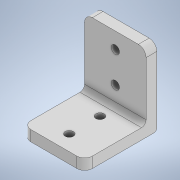
# Autodesk Inventor part: angulares
Saved by Autodesk Inventor 2022 (Build 260153000, 153)
## iProperties
Created: 2022-02-04
Part Number: angulares
Material: Generic
Document SubType Name: Modeling
Designer: Home
Density: 1 g/cm^3
Appearance: Default
Author: Home
Autodesk Inventor part; units mm, degrees
ref_plane "YZ Plane" through (0, 0, 0) normal (1, 0, 0) x (0, 1, 0)
ref_plane "XZ Plane" through (0, 0, 0) normal (0, 1, 0) x (-1, 0, 0)
ref_plane "XY Plane" through (0, 0, 0) normal (0, 0, 1) x (1, 0, 0)
sketch "Sketch1" plane through (0, 0, 0) normal (0, 1, 0) x (-1, 0, 0)
  line L0 (20, -20) -> (-20, -20)
  line L1 (-20, -20) -> (-20, 20)
  line L2 (-20, 20) -> (20, 20)
  line L3 (20, 20) -> (20, -20)
  line L4 (20, -20) -> (-20, 20) construction
  line L5 (-20, -20) -> (20, 20) construction
  point P0 (0, 0)
  dimension "d0" = 40
  dimension "d1" = 40
  constraints: 12 end point, 2 midpoint, 2 parallel, 1 horizontal, 1 perpendicular
  measures "d0" distance of L0.end L1.end
  measures "d1" distance of L0.start L0.end
extrude "Extrusion1" add sketch "Sketch1" along normal blind 7
sketch "Sketch2" plane through (0, 7, 0) normal (0, 1, 0) x (1, 0, 0)
  line L0 (-20, -20) -> (20, -20) projected
  point P0 (0, 0)
  point P1 (0, -10)
  point P2 (0, 10)
  dimension "d4" = 20
  dimension "d5" = 10
  constraints: 2 vertical alignment
  measures "d4" distance of point (0, 10) point (0, -10)
  measures "d5" distance from line of point (0, -10) L0
sketch "Sketch3" plane through (20, 0, -20) normal (0, 0, -1) x (-1, 0, 0)
  line L0 (0, 0) -> (0, 7) projected
  line L1 (0, 0) -> (40, 0)
  line L2 (40, 0) -> (40, 50)
  line L3 (40, 50) -> (0, 50)
  line L4 (0, 50) -> (0, 0)
  point P0 (20, 0)
  dimension "d14" = 50
  dimension "d15" = 40
  constraints: 8 end point, 2 parallel, 1 horizontal, 1 perpendicular
  measures "d14" distance of L3.end L0.start
  measures "d15" distance of L0.start L1.end
extrude "Extrusion2" add sketch "Sketch3" along normal blind 7
fillet "Fillet2" radius 3 1 edges at (0, 7, -20)
fillet "Fillet2" radius 5 4 edges at (-20, 50, -23.5) (20, 50, -23.5) (-20, 3.5, 20) (20, 3.5, 20)
fillet "Fillet2" radius 2 1 edges at (0, 0, -27)
sketch "Sketch4" plane through (20, 0, -20) normal (0, 0, 1) x (1, 0, 0)
  line L0 (-35, 0) -> (-5, 0) projected
  line L1 (-40, 7) -> (0, 7) projected
  point P0 (-20, 0)
  point P1 (-20, 39.5)
  point P2 (-20, 19.5)
  point P3 (-20, 0)
  point P4 (-20, 0)
  dimension "d22" = 20
  dimension "d23" = 12.5
  constraints: 2 midpoint, 2 vertical alignment
  measures "d22" distance of point (-20, 19.5) point (-20, 39.5)
  measures "d23" distance from line of point (-20, 19.5) L1
hole "Hole4" at (0, 39.5, -20) at (0, 19.5, -20) direction (0, 0, -1) diameter 5.4 end through all
hole "Hole5" at (0, 7, 10) at (0, 7, -10) direction (0, -1, 0) diameter 5.4 end through all
body "Solid1"
